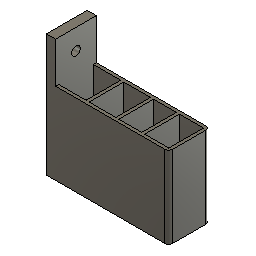
item40ToolHolder01 (Autodesk Fusion 360 design; units mm, degrees)
Autodesk Fusion 360 part; units mm, degrees
sketch "Sketch1" plane through (0, 0, 0) normal (0, 1, 0) x (1, 0, 0)
  line L0 (60, 20) -> (-60, 20)
  line L1 (-60, 20) -> (-60, -20)
  line L2 (-60, -20) -> (60, -20)
  line L3 (60, -20) -> (60, 20)
  line L4 (60, 20) -> (-60, -20) construction
  line L5 (-60, 20) -> (60, -20) construction
  line L6 (57, 17) -> (-57, 17)
  line L7 (-57, 17) -> (-57, -17)
  line L8 (-57, -17) -> (57, -17)
  line L9 (57, -17) -> (57, 17)
  line L10 (57, 17) -> (-57, -17) construction
  line L11 (-57, 17) -> (57, -17) construction
  line L12 (-24.159, 17) -> (-21.159, 17)
  line L13 (-21.159, 17) -> (-21.159, -17)
  line L14 (-21.159, -17) -> (-24.159, -17)
  line L15 (-24.159, -17) -> (-24.159, 17)
  line L16 (8.0431, 17) -> (8.0431, -17)
  line L17 (5.0431, -17) -> (5.0431, 17)
  line L18 (8.0431, -17) -> (5.0431, -17)
  line L19 (5.0431, 17) -> (8.0431, 17)
  line L20 (30.4518, 17) -> (33.4518, 17)
  line L21 (33.4518, 17) -> (33.4518, -17)
  line L22 (30.4518, -17) -> (30.4518, 17)
  line L23 (33.4518, -17) -> (30.4518, -17)
  dimension "d1" = 120
  dimension "d2" = 40
  dimension "d3" = 114
  dimension "d4" = 34
  dimension "d20" = 3
  dimension "d21" = 34
  dimension "d26" = 3
  dimension "d27" = 34
  dimension "d28" = 3
  dimension "d29" = 34
  constraint horizontal L0
  constraint perpendicular L0 L1
  constraint parallel L0 L2
  constraint parallel L1 L3
  constraint coincident L4 origin
  constraint coincident L5 origin
  constraint horizontal L6
  constraint perpendicular L6 L7
  constraint parallel L6 L8
  constraint parallel L7 L9
  constraint coincident L10 origin
  constraint coincident L11 origin
  constraint horizontal L12
  constraint vertical L13
  constraint horizontal L14
  constraint vertical L15
  constraint horizontal L19
  constraint vertical L16
  constraint horizontal L18
  constraint vertical L17
  constraint horizontal L20
  constraint vertical L21
  constraint horizontal L23
  constraint vertical L22
  constraint coincident L6 L12.start
  constraint coincident L6 L17.end
  constraint coincident L6 L20.start
  measures "d1" distance of L1.end L2.end
  measures "d2" distance of L0.end L1.end
  measures "d3" distance of L7.end L8.end
  measures "d4" distance of L6.end L7.end
  measures "d20" distance of L12.start L12.end
  measures "d21" distance of L12.start L14.end
  measures "d26" distance of L17.end L16.start
  measures "d27" distance of L17.start L17.end
  measures "d28" distance of L20.start L20.end
  measures "d29" distance of L22.start L20.start
extrude "Extrude1" add sketch "Sketch1" along normal blind 80 contours L0 L1 L2 L3 | L6 L8 L20 L21 L22 L23 | L6 L8 L16 L17 L18 L19 | L6 L8 L12 L13 L14 L15 makes body 1
extrude "Extrude2" add sketch "Sketch1" along normal blind 4 contours L6 L8 L9 L21 | L6 L8 L20 L21 L22 L23 | L6 L8 L16 L22 | L6 L8 L16 L17 L18 L19 | L6 L8 L13 L17 | L6 L8 L12 L13 L14 L15 | L6 L7 L8 L15 bodies 1
sketch "Sketch2" plane through (0, 0, 0) normal (1, 0, 0) x (0, 0, -1)
  line L0 (-20, 0) -> (20, 0)
  line L1 (20, 0) -> (20, 80)
  line L2 (20, 80) -> (-20, 80)
  line L3 (-20, 80) -> (-20, 0)
  line L4 (20, 120) -> (-20, 120)
  line L5 (-20, 120) -> (-20, 80)
  line L6 (-20, 80) -> (20, 80)
  line L7 (20, 80) -> (20, 120)
  line L8 (20, 120) -> (-20, 80) construction
  line L9 (-20, 120) -> (20, 80) construction
  line L10 (20, 0) -> (-20, 0)
  line L11 (-20, 0) -> (-20, -40)
  line L12 (-20, -40) -> (20, -40)
  line L13 (20, -40) -> (20, 0)
  line L14 (20, 0) -> (-20, -40) construction
  line L15 (-20, 0) -> (20, -40) construction
  circle A0 centre (0, 100) radius 4.25
  circle A1 centre (0, -20) radius 4.25
  point P0 (0, 100)
  point P1 (0, -20)
  dimension "d9" = 40
  dimension "d10" = 40
  dimension "d11" = 40
  dimension "d12" = 40
  dimension "d13" = 8.5
  dimension "d14" = 8.5
  constraint horizontal L4
  constraint perpendicular L4 L5
  constraint parallel L4 L6
  constraint parallel L5 L7
  constraint coincident L8 P0
  constraint coincident L9 P0
  constraint coincident L2.end L3.start
  constraint horizontal L10
  constraint perpendicular L10 L11
  constraint parallel L10 L12
  constraint parallel L11 L13
  constraint coincident L14 P1
  constraint coincident L15 P1
  constraint coincident L0.start L3.end
  constraint coincident P0 A0.centre
  constraint coincident P1 A1.centre
  measures "d9" distance of L2.end L1.end
  measures "d10" distance of L2.end L4.end
  measures "d11" distance of L11.end L12.end
  measures "d12" distance of L0.start L11.end
  measures "d13" diameter of A0
  measures "d14" diameter of A1
extrude "Extrude3" add sketch "Sketch2" along normal blind -60 and the other way blind 51 contours L0 L1 L2 L3 L6 L10 | L2 L4 L5 L6 L7 bodies 1
fillet "Fillet1" radius 4 2 edges at (60, 40, -20) (60, 40, 20) on bodies 1
copy_body "Body->Comp1" bodies 1 removing the originals makes body 2 in component "item40ToolHoplder-01"
component "item40ToolHoplder-01" placed x (1, 0, 0) y (0, 1, 0) z (0, 0, 1) at (0, 0, 0)
